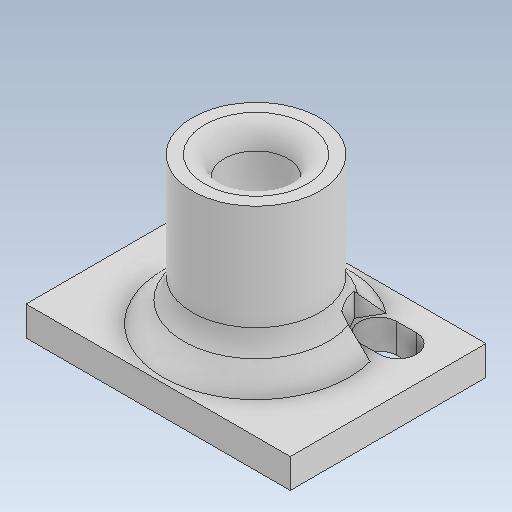
# Autodesk Inventor part: 11_Connettore_MPU
Saved by Autodesk Inventor 2020.2 (Build 242310000, 310)
## iProperties
Created: 2019-10-15
Part Number: 11_Connettore_MPU
Material: Generico
Document SubType Name: Modeling
Designer: socci
Density: 1 g/cm^3
Appearance: Default
Mass: 3.16762 g
Surface Area: 22.4279 cm^2
Volume: 3.16762 cm^3
Author: socci
Autodesk Inventor part; units mm, degrees
ref_plane "YZ Plane" through (0, 0, 0) normal (1, 0, 0) x (0, 1, 0)
ref_plane "XZ Plane" through (0, 0, 0) normal (0, 1, 0) x (-1, 0, 0)
ref_plane "XY Plane" through (0, 0, 0) normal (0, 0, 1) x (1, 0, 0)
sketch "Schizzo1" plane through (0, 0, 0) normal (0, 1, 0) x (-1, 0, 0)
  circle A0 centre (0, 0) radius 3.25
  circle A1 centre (0, 0) radius 6.5
  dimension "d0" = 6.5
  dimension "d1" = 13
  constraints: 2 centre point, 2 coincident
  measures "d0" diameter of A0
  measures "d1" diameter of A1
extrude "Estrusione1" add sketch "Schizzo1" along normal blind 15
sketch "Schizzo2" plane through (0, 0, 0) normal (0, -1, 0) x (1, 0, 0)
  line L0 (-13.5, -10) -> (13.5, -10)
  line L1 (13.5, -10) -> (13.5, 10)
  line L2 (13.5, 10) -> (-13.5, 10)
  line L3 (-13.5, 10) -> (-13.5, -10)
  line L4 (-13.5, -10) -> (13.5, 10) construction
  line L5 (13.5, -10) -> (-13.5, 10) construction
  point P0 (0, 0)
  point P1 (0, 0)
  point P2 (0, 0)
  dimension "d4" = 20
  dimension "d5" = 27
  constraints: 12 end point, 3 midpoint, 2 parallel, 1 coincident, 1 horizontal, 1 perpendicular
  measures "d4" distance of L2.end L0.start
  measures "d5" distance of L0.start L0.end
extrude "Estrusione2" add sketch "Schizzo2" along normal blind 3
sketch "Schizzo3" plane through (0, -3, 0) normal (0, -1, 0) x (1, 0, 0)
  line L0 (0, 0) -> (-8, 0)
  line L1 (0, 0) -> (8, 0) construction
  line L2 (-8, 0) -> (-8, -5.5)
  line L3 (0, 0) -> (8, 0)
  line L4 (0, 0) -> (8, 0) construction
  line L5 (8, 0) -> (8, -5.5)
  circle A0 centre (0, 0) radius 6.5 projected
  circle A1 centre (0, 0) radius 9.5 projected
  line L6 (-20.3813, -5.5) -> (-15.9716, -5.5)
  line L7 (-20.3813, -5.5) -> (-15.9716, -5.5) construction
  line L8 (-9, -5.5) -> (-7, -5.5)
  line L9 (-9, -5.5) -> (-7, -5.5) construction
  line L10 (-9, -5.5) -> (-7, -5.5) construction
  line L11 (-9, -7.4) -> (-7, -7.4)
  line L12 (-7, -3.6) -> (-9, -3.6)
  arc A2 (-9, -3.6) -> (-9, -7.4) centre (-9, -5.5) ccw
  arc A3 (-7, -7.4) -> (-7, -3.6) centre (-7, -5.5) ccw
  line L13 (7, -5.5) -> (9, -5.5)
  line L14 (7, -5.5) -> (9, -5.5) construction
  line L15 (7, -5.5) -> (9, -5.5) construction
  line L16 (7, -7.4) -> (9, -7.4)
  line L17 (9, -3.6) -> (7, -3.6)
  arc A4 (7, -3.6) -> (7, -7.4) centre (7, -5.5) ccw
  arc A5 (9, -7.4) -> (9, -3.6) centre (9, -5.5) ccw
  point P0 (2.8723, -8)
  point P1 (13.5, -10)
  point P2 (-13.5, -10)
  point P3 (8, -5.5)
  point P4 (0, -10)
  point P5 (0, 10)
  dimension "d21" = 8
  dimension "d22" = 180
  dimension "d23" = 5.5
  dimension "d24" = 90
  dimension "d25" = 8
  dimension "d26" = 0
  dimension "d27" = 5.5
  dimension "d28" = 90
  dimension "d31" = 0
  dimension "d32" = 0
  dimension "d33" = 2
  dimension "d34" = 3.8
  dimension "d35" = 0
  dimension "d36" = 3.8
  dimension "d37" = 2
  constraints: 40 end point, 8 horizontal, 8 point on circle, 8 tangent, 5 collinear, 4 centre point, 4 midpoint, 3 equal length, 2 perpendicular, 1 other
  measures "d21" distance of L0.start L0.end
  measures "d22" angle of L0 L1
  measures "d23" distance of L2.end L0.end
  measures "d24" angle of L2 L0
  measures "d25" distance of L0.start L1.end
  measures "d26" distance between parallel lines of L3 L4
  measures "d27" distance of L5.end L1.end
  measures "d28" angle of L3 L5
  measures "d31" distance between parallel lines of L6 L7
  measures "d32" distance between parallel lines of L8 L9
  measures "d33" distance of L8.start L9.end
  measures "d34" diameter of A3
  measures "d35" distance between parallel lines of L13 L14
  measures "d36" diameter of A5
  measures "d37" distance of L13.start L13.end
extrude "Estrusione3" cut sketch "Schizzo3" against normal blind 10 contours L12 A3 A1 L2 | L2 A1 L12 | L17 A1 L5 | L5 A1 A4 L17 | A1 L8 L2 | L2 L8 A1 A3 L11 A2 L12 | A1 L17 A5 L16 A4 L13 L5 | L5 L13 A1
fillet "Raccordo2" radius 2 1 edges at (3.25, 15, 0)
chamfer "Smusso2" distance 3 angle 45 1 edges at (6.5, 0, 0) measured on face at (7, 0, 0)
fillet "Raccordo3" radius 3 1 edges at (6.5, 3, 0)
sketch "Schizzo4" plane through (0, 0, 0) normal (0, 1, 0) x (1, 0, 0)
  arc A0 (9, 3.6) -> (9, 7.4) centre (9, 5.5) ccw projected
  arc A1 (7, 7.4) -> (7, 3.6) centre (7, 5.5) ccw projected
  line L0 (9, 5.5) -> (7, 5.5)
  arc A2 (-9, 7.4) -> (-9, 3.6) centre (-9, 5.5) ccw projected
  arc A3 (-7, 3.6) -> (-7, 7.4) centre (-7, 5.5) ccw projected
  line L1 (-9, 5.5) -> (-7, 5.5)
  circle A4 centre (8, 5.5) radius 3
  circle A5 centre (-8, 5.5) radius 3
  line L2 (6.2679, 2.5) -> (4.5359, 5.5)
  line L3 (4.5359, 5.5) -> (6.2679, 8.5)
  line L4 (6.2679, 8.5) -> (9.7321, 8.5)
  line L5 (9.7321, 8.5) -> (11.4641, 5.5)
  line L6 (11.4641, 5.5) -> (9.7321, 2.5)
  line L7 (9.7321, 2.5) -> (6.2679, 2.5)
  line L8 (-6.2679, 8.5) -> (-4.5359, 5.5)
  line L9 (-4.5359, 5.5) -> (-6.2679, 2.5)
  line L10 (-6.2679, 2.5) -> (-9.7321, 2.5)
  line L11 (-9.7321, 2.5) -> (-11.4641, 5.5)
  line L12 (-11.4641, 5.5) -> (-9.7321, 8.5)
  line L13 (-9.7321, 8.5) -> (-6.2679, 8.5)
  point P0 (0, 0)
  point P1 (9.3191, 3.627)
  point P2 (-9.3191, 3.627)
  point P3 (8, 2.5)
  point P4 (-8, 8.5)
  dimension "d45" = 6
  dimension "d46" = 6
  constraints: 28 end point, 4 midpoint, 3 coincident, 2 horizontal, 2 vertical alignment, 30 other
extrude "Estrusione6" cut sketch "Schizzo4" along normal blind 6
